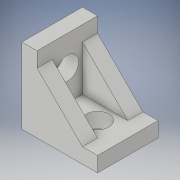
# Autodesk Inventor part: Base auxiliar - esquadra
Saved by Autodesk Inventor 2019 (Build 230136000, 136)
## iProperties
Created: 2018-09-12
Part Number: Base auxiliar - esquadra
Material: Genérico
Document SubType Name: Modeling
Designer: Albert Garangou Culebras
Density: 1 g/cm^3
Appearance: Valor por defecto
Author: Albert Garangou Culebras
Autodesk Inventor part; units mm, degrees
ref_plane "YZ Plane" through (0, 0, 0) normal (1, 0, 0) x (0, 1, 0)
ref_plane "XZ Plane" through (0, 0, 0) normal (0, 1, 0) x (-1, 0, 0)
ref_plane "XY Plane" through (0, 0, 0) normal (0, 0, 1) x (1, 0, 0)
sketch "Boceto1" plane through (0, 0, 0) normal (0, 1, 0) x (-1, 0, 0)
  circle A0 centre (0, 0) radius 1.5
  line L0 (4, 4) -> (-4, 4)
  line L1 (-4, 4) -> (-4, -4)
  line L2 (-4, -4) -> (4, -4)
  line L3 (4, -4) -> (4, 4)
  dimension "d0" = 3
  constraints: 8 end point, 2 parallel, 1 centre point, 1 coincident, 1 horizontal, 1 perpendicular
  measures "d0" diameter of A0
extrude "Extrusión1" add sketch "Boceto1" along normal blind 2
sketch "Boceto2" plane through (-4, 0, -4) normal (-1, 0, 0) x (0, 0, 1)
  circle A0 centre (4, 6) radius 1.5
  line L0 (8, 2) -> (8, 10)
  line L1 (8, 10) -> (0, 10)
  line L2 (0, 10) -> (0, 2)
  line L3 (8, 0) -> (0, 0) projected
  line L4 (0, 0) -> (8, 0)
  line L5 (8, 0) -> (8, 2)
  line L6 (0, 2) -> (0, 0)
  line L7 (0, 0) -> (8, 0)
  line L8 (8, 0) -> (8, 10)
  line L9 (8, 10) -> (0, 10)
  line L10 (0, 10) -> (0, 0)
  point P0 (4, 0)
  constraints: 20 end point, 4 parallel, 2 horizontal, 2 perpendicular, 1 centre point
extrude "Extrusión2" add sketch "Boceto2" along normal blind 2
sketch "Boceto3" plane through (4, 0, 4) normal (0, 0, 1) x (1, 0, 0)
  line L0 (-8, 2) -> (-8, 10) projected
  line L1 (-8, 10) -> (-8, 8)
  line L2 (0, 2) -> (-2, 2)
  line L3 (-2, 2) -> (-8, 8)
  line L4 (-2, 2) -> (-8, 2)
  line L5 (-8, 8) -> (-8, 2)
  point P0 (-5.5, 2)
  point P1 (-8, 4.5)
  dimension "d26" = 2
  dimension "d27" = 2
  constraints: 10 end point, 2 horizontal, 1 collinear, 1 point on line
  measures "d26" distance of L0.end L1.end
  measures "d27" distance of L2.start L2.end
extrude "Extrusión8" add sketch "Boceto3" against normal blind 2
sketch "Boceto9" plane through (4, 0, -4) normal (0, 0, -1) x (-1, 0, 0)
  line L0 (0, 2) -> (8, 2) projected
  line L1 (8, 8) -> (2, 2) projected
  line L2 (2, 2) -> (8, 8)
  line L3 (8, 8) -> (8, 2)
  line L4 (8, 2) -> (2, 2)
  point P0 (4, 0)
  constraints: 6 end point, 1 collinear, 1 perpendicular, 1 point on line, 1 vertical
extrude "Extrusión9" add sketch "Boceto9" against normal blind 2
